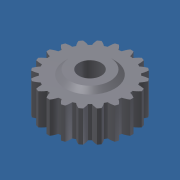
# Autodesk Inventor part: Stirnzahnrad2
Saved by Autodesk Inventor 2014 SP2 (Build 180246200, 246)
## iProperties
Created: 2015-01-19
Part Number: Stirnzahnrad2
Material: Steel
Document SubType Name: Modeling
Designer: 4ndreas
Categories: <?xml version="1.0" encoding="UTF-16"?> <MemberInstance><Categories><FamilyTemplate><FamilyTemplateParameter ValueType="xs:double" Id="1" ObjectReferenceKey="da_z" ObjectType="kUserParameterObject"/><FamilyTemplateParameter ValueType="xs:double" Id="2" ObjectReferenceKey="da_b" ObjectType="kUserParameterObject"/><FamilyTemplateParameter ValueType="xs:double" Id="3" ObjectReferenceKey="da_beta" ObjectType="kUserParameterObject"/><FamilyTemplateParameter ValueType="xs:double" Id="4" ObjectReferenceKey="da_da" ObjectType="kUserParameterObject"/><FamilyTemplateParameter ValueType="xs:double" Id="5" ObjectReferenceKey="da_aw" ObjectType="kUserParameterObject"/><FamilyTemplateParameter ValueType="xs:string" Id="6" ObjectReferenceKey="EAIAABAAAACIAQAAAAAAAIAAAAAAAAAA" ObjectType="83910656" SubObjectId="SurfaceGeometry"/></FamilyTemplate><ParamToTemplateMap><ParamToTemplate CategoryParameter="//CategoryParameter[@InternalName='046C89C9-8512-4d59-83FE-43B91F4F132A']" TemplateParameter="1"/><ParamToTemplate CategoryParameter="//CategoryParameter[@InternalName='2552DF32-E462-4b46-AEBF-C6C7768E72AC']" TemplateParameter="2"/><ParamToTemplate CategoryParameter="//CategoryParameter[@InternalName='C9EE641D-15FC-4fae-A226-E94C4372FDD7']" TemplateParameter="3"/><ParamToTemplate><ParamToTemplate CategoryParameter="//CategoryParameter[@InternalName='00B6519A-459B-49c7-AD84-2E56D39A5744']" ConstantValue="0.764508"/></ParamToTemplate><ParamToTemplate><ParamToTemplate CategoryParameter="//CategoryParameter[@InternalName='04B31F0E-C7A6-4894-AA32-9629BEFACF47']" ConstantValue="1.000000"/></ParamToTemplate><ParamToTemplate><ParamToTemplate CategoryParameter="//CategoryParameter[@InternalName='43CBEC2E-7847-49e7-A936-2F7889FCB2D9']" ConstantValue="0.250000"/></ParamToTemplate><ParamToTemplate><ParamToTemplate CategoryParameter="//CategoryParameter[@InternalName='B1EFC894-105D-4ebd-86BF-FA20ED196853']" ConstantValue="0.302500"/></ParamToTemplate><ParamToTemplate><ParamToTemplate CategoryParameter="//CategoryParameter[@InternalName='51175063-3D10-4879-93E8-6246FE8B403D']" ConstantValue="2060000000.000000"/></ParamToTemplate><ParamToTemplate><ParamToTemplate CategoryParameter="//CategoryParameter[@InternalName='A3A52E27-4454-46a9-B0BD-C932399B70AF']" ConstantValue="0.300000"/></ParamToTemplate><ParamToTemplate><ParamToTemplate CategoryParameter="//CategoryParameter[@InternalName='91B76062-C214-41d9-B1B9-14D2AB99603D']" ConstantValue="0.085000"/></ParamToTemplate><ParamToTemplate><ParamToTemplate CategoryParameter="//CategoryParameter[@InternalName='374E806E-8B8A-4dda-A9AA-1039D6500AD2']" ConstantValue="11.764706"/></ParamToTemplate><ParamToTemplate><ParamToTemplate CategoryParameter="//CategoryParameter[@InternalName='2D373A89-B862-43d6-8D0B-0CBF12AB9F6C']" ConstantValue="0.174533"/></ParamToTemplate><ParamToTemplate CategoryParameter="//CategoryParameter[@InternalName='37777632-D6A2-4fac-9D53-DB8ACD95C989']" TemplateParameter="4"/><ParamToTemplate CategoryParameter="//CategoryParameter[@InternalName='FD1017F1-B727-4f7e-9707-0F86F1FF9423']" TemplateParameter="5"/><ParamToTemplate><ParamToTemplate CategoryParameter="//CategoryParameter[@InternalName='9E1B4470-B2D3-4ff1-B813-535BB4CDF51A']" ConstantValue="3520000.000000"/></ParamToTemplate><ParamToTemplate><ParamToTemplate CategoryParameter="//CategoryParameter[@InternalName='F8452263-BFF6-458c-9FB1-07C4B99E95CD']" ConstantValue="11400000.000000"/></ParamToTemplate><ParamToTemplate><ParamToTemplate CategoryParameter="//CategoryParameter[@InternalName='3E3BB259-FD49-497f-8171-6EBC954A3479']" ConstantValue="2.000000"/></ParamToTemplate><ParamToTemplate CategoryParameter="//CategoryParameter[@InternalName='27C3BAF2-7550-4e4b-AE2C-0DB134B7D9B7']" TemplateParameter="6"/></ParamToTemplateMap><Category DisplayName="Gear" InternalName="DC85795E-93AB-48d5-8EEE-5A27447B64BD" Mnemonic="Gear"><CategoryParameter DisplayName="z" InternalName="046C89C9-8512-4d59-83FE-43B91F4F132A" Mnemonic="z"/><CategoryParameter DisplayName="b" InternalName="2552DF32-E462-4b46-AEBF-C6C7768E72AC" Mnemonic="b"/><CategoryParameter DisplayName="||b|" InternalName="C9EE641D-15FC-4fae-A226-E94C4372FDD7" Mnemonic="beta"/><CategoryParameter DisplayName="x" InternalName="00B6519A-459B-49c7-AD84-2E56D39A5744" Mnemonic="x"/><CategoryParameter DisplayName="a*" InternalName="04B31F0E-C7A6-4894-AA32-9629BEFACF47" Mnemonic="a"/><CategoryParameter DisplayName="c*" InternalName="43CBEC2E-7847-49e7-A936-2F7889FCB2D9" Mnemonic="c"/><CategoryParameter DisplayName="r|.f|*" InternalName="B1EFC894-105D-4ebd-86BF-FA20ED196853" Mnemonic="rf"/><CategoryParameter DisplayName="E" InternalName="51175063-3D10-4879-93E8-6246FE8B403D" Mnemonic="E"/><CategoryParameter DisplayName="||m|" InternalName="A3A52E27-4454-46a9-B0BD-C932399B70AF" Mnemonic="mi"/><Category DisplayName="SpurGear" InternalName="26C5A22E-A91E-4dfd-A3B3-23CCAFAE1764" Mnemonic="SpurGear"><CategoryParameter DisplayName="m" InternalName="91B76062-C214-41d9-B1B9-14D2AB99603D" Mnemonic="m"/><CategoryParameter DisplayName="P" InternalName="374E806E-8B8A-4dda-A9AA-1039D6500AD2" Mnemonic="PP"/><CategoryParameter DisplayName="||a|" InternalName="2D373A89-B862-43d6-8D0B-0CBF12AB9F6C" Mnemonic="alpha"/><CategoryParameter DisplayName="d|.a|" InternalName="37777632-D6A2-4fac-9D53-DB8ACD95C989" Mnemonic="da"/><CategoryParameter DisplayName="a|.w|" InternalName="FD1017F1-B727-4f7e-9707-0F86F1FF9423" Mnemonic="aw"/><CategoryParameter DisplayName="||s||.Flim|" InternalName="9E1B4470-B2D3-4ff1-B813-535BB4CDF51A" Mnemonic="sFlim"/><CategoryParameter DisplayName="||s||.Hlim|" InternalName="F8452263-BFF6-458c-9FB1-07C4B99E95CD" Mnemonic="sHlim"/><CategoryParameter DisplayName="Typ" InternalName="3E3BB259-FD49-497f-8171-6EBC954A3479" Mnemonic="type"/><CategoryParameter DisplayName="PitchDiameter" InternalName="27C3BAF2-7550-4e4b-AE2C-0DB134B7D9B7" Mnemonic="IDS_PITCHDIAM"/></Category></Category></Categories></MemberInstance>
Density: 1 g/cm^3
Appearance: Steel
CustomPartVersion: 1
Author: 4ndreas
Autodesk Inventor part; units mm, degrees
sketch "Sketch1" plane through (0, 0, 0) normal (0, 0, 1) x (1, 0, 0)
  circle A0 centre (0, 0) radius 9.3602
  dimension "d0" = 18.7203
  constraints: 1 centre point
  measures "d0" diameter of A0
extrude "Extrusion1" add sketch "Sketch1" along normal blind 7
ref_plane "Work Plane2" through (0, 0, 3.5) normal (0, 0, 1) x (1, 0, 0)
sketch "Sketch2" plane through (0, 0, 0) normal (0, 0, -1) x (-1, 0, 0)
  circle A0 centre (0, 0) radius 9.3602 projected
  circle A1 centre (0, 0) radius 9
  dimension "d3" = 18
  constraints: 1 centre point, 1 coincident
  measures "d3" diameter of A1
surface extrude "Flankendurchmesser" sketch "Sketch2" against normal through all shown no curves A1
ref_plane "Work Plane8" through (0, 0, 0) normal (0.9876883, 0.1564345, 0) x (0, 0, 1)
ref_plane "Work Plane9" through (0, 0, 0) normal (1, 0, 0) x (0, 1, 0)
spur gear teeth "Stirnzahnrad" teeth 20 pitch diameter 17 tip diameter 18.7203 root diameter 16.1747 face width 7 start plane through (0, 0, 0) normal (0, 0, -1) x (-1, 0, 0)
sketch "Skizze3" plane through (0, 0, 7) normal (0, 0, 1) x (1, 0, 0)
  arc A0 (-3.3858, 7.3445) -> (-3.9516, 7.0562) centre (0, 0) ccw projected
hole "Bohrung1" at (0, 0, 7) direction (0, 0, -1) diameter 5 end through all
sketch "Skizze4" plane through (0, 0, 0) normal (0, 0, -1) x (-1, 0, 0)
  circle A0 centre (0, 0) radius 3.5
  arc A1 (-2.5407, 9.0087) -> (-3.2397, 8.7816) centre (0, 0) ccw
  line L0 (-2.3094, 4) -> (2.3094, 4)
  line L1 (2.3094, 4) -> (4.6188, 0)
  line L2 (4.6188, 0) -> (2.3094, -4)
  line L3 (2.3094, -4) -> (-2.3094, -4)
  line L4 (-2.3094, -4) -> (-4.6188, 0)
  line L5 (-4.6188, 0) -> (-2.3094, 4)
  circle A2 centre (0, 0) radius 2.5 projected
  arc A3 (3.3858, 7.3445) -> (3.2397, 8.7816) centre (-1.0508, 7.6194) ccw projected
  arc A4 (3.2397, 8.7816) -> (2.5407, 9.0087) centre (0, 0) ccw projected
  arc A5 (2.5407, 9.0087) -> (1.5778, 7.9319) centre (5.3287, 5.5465) ccw projected
  arc A6 (1.5778, 7.9319) -> (0.9506, 8.0313) centre (0, 0) ccw projected
  arc A7 (0.9506, 8.0313) -> (0.3675, 9.353) centre (-3.3539, 6.9217) ccw projected
  arc A8 (0.3675, 9.353) -> (-0.3675, 9.353) centre (0, 0) ccw projected
  arc A9 (-0.3675, 9.353) -> (-0.9506, 8.0313) centre (3.3539, 6.9217) ccw projected
  arc A10 (-0.9506, 8.0313) -> (-1.5778, 7.9319) centre (0, 0) ccw projected
  arc A11 (-1.5778, 7.9319) -> (-2.5407, 9.0087) centre (-5.3287, 5.5465) ccw projected
  arc A12 (-2.5407, 9.0087) -> (-3.2397, 8.7816) centre (0, 0) ccw projected
  arc A13 (-3.2397, 8.7816) -> (-3.3858, 7.3445) centre (1.0508, 7.6194) ccw projected
  arc A14 (-3.3858, 7.3445) -> (-3.9516, 7.0562) centre (0, 0) ccw projected
  arc A15 (-3.9516, 7.0562) -> (-5.2002, 7.7827) centre (-6.7819, 3.6284) ccw projected
  arc A16 (-5.2002, 7.7827) -> (-5.7948, 7.3507) centre (0, 0) ccw projected
  arc A17 (-5.7948, 7.3507) -> (-5.4897, 5.9387) centre (-1.3551, 7.5712) ccw projected
  arc A18 (-5.4897, 5.9387) -> (-5.9387, 5.4897) centre (0, 0) ccw projected
  arc A19 (-5.9387, 5.4897) -> (-7.3507, 5.7948) centre (-7.5712, 1.3551) ccw projected
  arc A20 (-7.3507, 5.7948) -> (-7.7827, 5.2002) centre (0, 0) ccw projected
  arc A21 (-7.7827, 5.2002) -> (-7.0562, 3.9516) centre (-3.6284, 6.7819) ccw projected
  arc A22 (-7.0562, 3.9516) -> (-7.3445, 3.3858) centre (0, 0) ccw projected
  arc A23 (-7.3445, 3.3858) -> (-8.7816, 3.2397) centre (-7.6194, -1.0508) ccw projected
  arc A24 (-8.7816, 3.2397) -> (-9.0087, 2.5407) centre (0, 0) ccw projected
  arc A25 (-9.0087, 2.5407) -> (-7.9319, 1.5778) centre (-5.5465, 5.3287) ccw projected
  arc A26 (-7.9319, 1.5778) -> (-8.0313, 0.9506) centre (0, 0) ccw projected
  arc A27 (-8.0313, 0.9506) -> (-9.353, 0.3675) centre (-6.9217, -3.3539) ccw projected
  arc A28 (-9.353, 0.3675) -> (-9.353, -0.3675) centre (0, 0) ccw projected
  arc A29 (-9.353, -0.3675) -> (-8.0313, -0.9506) centre (-6.9217, 3.3539) ccw projected
  arc A30 (-8.0313, -0.9506) -> (-7.9319, -1.5778) centre (0, 0) ccw projected
  arc A31 (-7.9319, -1.5778) -> (-9.0087, -2.5407) centre (-5.5465, -5.3287) ccw projected
  arc A32 (-9.0087, -2.5407) -> (-8.7816, -3.2397) centre (0, 0) ccw projected
  arc A33 (-8.7816, -3.2397) -> (-7.3445, -3.3858) centre (-7.6194, 1.0508) ccw projected
  arc A34 (-7.3445, -3.3858) -> (-7.0562, -3.9516) centre (0, 0) ccw projected
  arc A35 (-7.0562, -3.9516) -> (-7.7827, -5.2002) centre (-3.6284, -6.7819) ccw projected
  arc A36 (-7.7827, -5.2002) -> (-7.3507, -5.7948) centre (0, 0) ccw projected
  arc A37 (-7.3507, -5.7948) -> (-5.9387, -5.4897) centre (-7.5712, -1.3551) ccw projected
  arc A38 (-5.9387, -5.4897) -> (-5.4897, -5.9387) centre (0, 0) ccw projected
  arc A39 (-5.4897, -5.9387) -> (-5.7948, -7.3507) centre (-1.3551, -7.5712) ccw projected
  arc A40 (-5.7948, -7.3507) -> (-5.2002, -7.7827) centre (0, 0) ccw projected
  arc A41 (-5.2002, -7.7827) -> (-3.9516, -7.0562) centre (-6.7819, -3.6284) ccw projected
  arc A42 (-3.9516, -7.0562) -> (-3.3858, -7.3445) centre (0, 0) ccw projected
  arc A43 (-3.3858, -7.3445) -> (-3.2397, -8.7816) centre (1.0508, -7.6194) ccw projected
  arc A44 (-3.2397, -8.7816) -> (-2.5407, -9.0087) centre (0, 0) ccw projected
  arc A45 (-2.5407, -9.0087) -> (-1.5778, -7.9319) centre (-5.3287, -5.5465) ccw projected
  arc A46 (-1.5778, -7.9319) -> (-0.9506, -8.0313) centre (0, 0) ccw projected
  arc A47 (-0.9506, -8.0313) -> (-0.3675, -9.353) centre (3.3539, -6.9217) ccw projected
  arc A48 (-0.3675, -9.353) -> (0.3675, -9.353) centre (0, 0) ccw projected
  arc A49 (0.3675, -9.353) -> (0.9506, -8.0313) centre (-3.3539, -6.9217) ccw projected
  arc A50 (0.9506, -8.0313) -> (1.5778, -7.9319) centre (0, 0) ccw projected
  arc A51 (1.5778, -7.9319) -> (2.5407, -9.0087) centre (5.3287, -5.5465) ccw projected
  arc A52 (2.5407, -9.0087) -> (3.2397, -8.7816) centre (0, 0) ccw projected
  arc A53 (3.2397, -8.7816) -> (3.3858, -7.3445) centre (-1.0508, -7.6194) ccw projected
  arc A54 (3.3858, -7.3445) -> (3.9516, -7.0562) centre (0, 0) ccw projected
  arc A55 (3.9516, -7.0562) -> (5.2002, -7.7827) centre (6.7819, -3.6284) ccw projected
  arc A56 (5.2002, -7.7827) -> (5.7948, -7.3507) centre (0, 0) ccw projected
  arc A57 (5.7948, -7.3507) -> (5.4897, -5.9387) centre (1.3551, -7.5712) ccw projected
  arc A58 (5.4897, -5.9387) -> (5.9387, -5.4897) centre (0, 0) ccw projected
  arc A59 (5.9387, -5.4897) -> (7.3507, -5.7948) centre (7.5712, -1.3551) ccw projected
  arc A60 (7.3507, -5.7948) -> (7.7827, -5.2002) centre (0, 0) ccw projected
  arc A61 (7.7827, -5.2002) -> (7.0562, -3.9516) centre (3.6284, -6.7819) ccw projected
  arc A62 (7.0562, -3.9516) -> (7.3445, -3.3858) centre (0, 0) ccw projected
  arc A63 (7.3445, -3.3858) -> (8.7816, -3.2397) centre (7.6194, 1.0508) ccw projected
  arc A64 (8.7816, -3.2397) -> (9.0087, -2.5407) centre (0, 0) ccw projected
  arc A65 (9.0087, -2.5407) -> (7.9319, -1.5778) centre (5.5465, -5.3287) ccw projected
  arc A66 (7.9319, -1.5778) -> (8.0313, -0.9506) centre (0, 0) ccw projected
  arc A67 (8.0313, -0.9506) -> (9.353, -0.3675) centre (6.9217, 3.3539) ccw projected
  arc A68 (9.353, -0.3675) -> (9.353, 0.3675) centre (0, 0) ccw projected
  arc A69 (9.353, 0.3675) -> (8.0313, 0.9506) centre (6.9217, -3.3539) ccw projected
  arc A70 (8.0313, 0.9506) -> (7.9319, 1.5778) centre (0, 0) ccw projected
  arc A71 (7.9319, 1.5778) -> (9.0087, 2.5407) centre (5.5465, 5.3287) ccw projected
  arc A72 (9.0087, 2.5407) -> (8.7816, 3.2397) centre (0, 0) ccw projected
  arc A73 (8.7816, 3.2397) -> (7.3445, 3.3858) centre (7.6194, -1.0508) ccw projected
  arc A74 (7.3445, 3.3858) -> (7.0562, 3.9516) centre (0, 0) ccw projected
  arc A75 (7.0562, 3.9516) -> (7.7827, 5.2002) centre (3.6284, 6.7819) ccw projected
  arc A76 (7.7827, 5.2002) -> (7.3507, 5.7948) centre (0, 0) ccw projected
  arc A77 (7.3507, 5.7948) -> (5.9387, 5.4897) centre (7.5712, 1.3551) ccw projected
  arc A78 (5.9387, 5.4897) -> (5.4897, 5.9387) centre (0, 0) ccw projected
  arc A79 (5.4897, 5.9387) -> (5.7948, 7.3507) centre (1.3551, 7.5712) ccw projected
  arc A80 (5.7948, 7.3507) -> (5.2002, 7.7827) centre (0, 0) ccw projected
  arc A81 (5.2002, 7.7827) -> (3.9516, 7.0562) centre (6.7819, 3.6284) ccw projected
  arc A82 (3.9516, 7.0562) -> (3.3858, 7.3445) centre (0, 0) ccw projected
  dimension "d56" = 8
  constraints: 12 end point, 2 centre point, 2 point on circle, 1 coincident, 1 horizontal, 13 other
  measures "d56" distance between parallel lines of L3 L0
extrude "Extrusion2" cut sketch "Skizze4" against normal blind 3 contours A0 | L0 L1 L2 L3 L4 L5 | A2
sketch "Skizze5" plane through (0, 0, 7) normal (0, 0, 1) x (1, 0, 0)
  circle A0 centre (0, 0) radius 2.5 projected
  arc A1 (-2.5407, 9.0087) -> (-3.2397, 8.7816) centre (0, 0) ccw projected
  circle A2 centre (0, 0) radius 5.5
  dimension "d59" = 3
  constraints: 1 centre point, 1 coincident
  measures "d59" radial gap between concentric circles of A2 A0
extrude "Extrusion3" add sketch "Skizze5" along normal blind 1
chamfer "Fase1" distance 1 angle 45 1 edges at (-5.5, 0, 8)
equation "\"d0\" = da_da"
equation "\"d1\" = da_b"
equation "\"d3\" = da_dw"
equation "\"d16\" = da_aw"
equation "\"d43\" = da_aw"
equation "\"d46\" = da_aw"
equation "\"da_da\" = 18.720336"
equation "\"da_b\" = 7"
equation "\"da_dw\" = 18"
equation "\"da_aw\" = 18"
body "Solid1"
body "Srf1"
